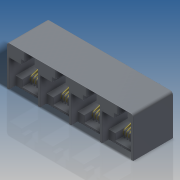
# Autodesk Inventor part: 11035-LtBluishGray
Saved by Autodesk Inventor 2016 SP2 (Build 200236200, 236)
## iProperties
Created: 2015-08-19
Part Number: 11035-LtBluishGray
Material: ABS Plastic
Document SubType Name: Modeling
Designer: D. Kohfeld
Density: 1.06 g/cm^3
Appearance: LtBluishGray
Mass: 4.59021 g
Surface Area: 62.0257 cm^2
Volume: 4.33039 cm^3
Author: D. Kohfeld
Autodesk Inventor part; units mm, degrees
ref_plane "XZ Plane" through (0, 0, 0) normal (0, 1, 0) x (-1, 0, 0)
ref_plane "XY Plane" through (0, 0, 0) normal (0, 0, 1) x (1, 0, 0)
sketch "Sketch2" plane through (0, 0, 0) normal (0, 0, 1) x (1, 0, 0)
  line L0 (-22.8, -6.8) -> (-22.8, 6.8)
  arc A0 (-21.84, 7.76) -> (-22.8, 6.8) centre (-21.84, 6.8) ccw
  line L1 (-21.84, 7.76) -> (21.84, 7.76)
  arc A1 (22.8, 6.8) -> (21.84, 7.76) centre (21.84, 6.8) ccw
  line L2 (22.8, 6.8) -> (22.8, -6.8)
  line L3 (22.8, -6.8) -> (-22.8, -6.8)
  line L4 (-22, -6.8) -> (-22, 3.2)
  line L5 (-22, 3.2) -> (-17.6, 3.2)
  line L6 (-17.6, 3.2) -> (-17.6, 4.8)
  line L7 (-17.6, 4.8) -> (-16.4, 4.8)
  line L8 (-16.4, 4.8) -> (-16.4, 6.8)
  line L9 (-16.4, 6.8) -> (-12.8, 6.8)
  line L10 (-12.8, 6.8) -> (-12.8, 4.8)
  line L11 (-12.8, 4.8) -> (-11.6, 4.8)
  line L12 (-11.6, 4.8) -> (-11.6, -6.8)
  line L13 (-22, -3.6) -> (-19.6, -3.6)
  line L14 (-19.6, -3.6) -> (-19.6, -6)
  line L15 (-19.6, -6) -> (-19, -6)
  line L16 (-19, -6) -> (-18.6, -6)
  line L17 (-18.6, -6) -> (-18, -6)
  line L18 (-18, -6) -> (-17.6, -6)
  line L19 (-17.6, -6) -> (-17, -6)
  line L20 (-17, -6) -> (-16.6, -6)
  line L21 (-16.6, -6) -> (-16, -6)
  line L22 (-16, -6) -> (-15.6, -6)
  line L23 (-15.6, -6) -> (-15, -6)
  line L24 (-15, -6) -> (-14.6, -6)
  line L25 (-14.6, -6) -> (-14, -6)
  line L26 (-14, -6) -> (-14, -3.6)
  line L27 (-14, -3.6) -> (-11.6, -3.6)
  line L28 (-19, -6) -> (-19, -3.6)
  line L29 (-18.6, -6) -> (-18.6, -3.6)
  line L30 (-18, -6) -> (-18, -3.6)
  line L31 (-17.6, -6) -> (-17.6, -3.6)
  line L32 (-17, -6) -> (-17, -3.6)
  line L33 (-16.6, -6) -> (-16.6, -3.6)
  line L34 (-16, -6) -> (-16, -3.6)
  line L35 (-15.6, -6) -> (-15.6, -3.6)
  line L36 (-15, -6) -> (-15, -3.6)
  line L37 (-14.6, -6) -> (-14.6, -3.6)
  line L38 (-19.6, -3.6) -> (-19, -3.6)
  line L39 (-19, -3.6) -> (-18.6, -3.6)
  line L40 (-18.6, -3.6) -> (-18, -3.6)
  line L41 (-18, -3.6) -> (-17.6, -3.6)
  line L42 (-17.6, -3.6) -> (-17, -3.6)
  line L43 (-17, -3.6) -> (-16.6, -3.6)
  line L44 (-16.6, -3.6) -> (-16, -3.6)
  line L45 (-16, -3.6) -> (-15.6, -3.6)
  line L46 (-15.6, -3.6) -> (-15, -3.6)
  line L47 (-15, -3.6) -> (-14.6, -3.6)
  line L48 (-14.6, -3.6) -> (-14, -3.6)
  line L49 (-17.6, 4.8) -> (-17.6, 6.8)
  line L50 (-17.6, 6.8) -> (-16.4, 6.8)
  line L51 (-12.8, 6.8) -> (-11.6, 6.8)
  line L52 (-11.6, 6.8) -> (-11.6, 4.8)
  point P0 (0, 0)
  point P1 (0, 7.76)
  point P2 (-22.8, 0)
  dimension "d0" = 45.6
  dimension "d1" = 14.56
  dimension "d2" = 0.96
  dimension "d3" = 10.4
  dimension "d4" = 0.96
  dimension "d5" = 3.6
  dimension "d6" = 6
  dimension "d8" = 2
  dimension "d9" = 1.6
  dimension "d10" = 0.8
  dimension "d11" = 3.2
  dimension "d12" = 2.4
  dimension "d13" = 0.4
  dimension "d14" = 5.6
  constraints: 106 end point, 32 horizontal, 21 vertical, 11 collinear, 4 point on circle, 4 point on line, 4 tangent, 2 centre point, 2 horizontal alignment, 2 midpoint, 1 equal radius, 1 vertical alignment
  measures "d0" distance between parallel lines of L0 L2
  measures "d1" distance between parallel lines of L3 L1
  measures "d2" radius of A0
  measures "d3" distance between parallel lines of L12 L4
  measures "d4" distance between parallel lines of L1 L9
  measures "d5" distance of L8.end L9.end
  measures "d6" distance between parallel lines of L12 L6
  measures "d8" distance of L7.end L8.end
  measures "d9" distance of L5.end L6.end
  measures "d10" distance between parallel lines of L0 L4
  measures "d11" distance between parallel lines of L3 L13
  measures "d12" distance of L13.end L14.end
  measures "d13" distance between parallel lines of L29 L28
  measures "d14" distance between parallel lines of L26 L14
extrude "Extrusion1" add sketch "Sketch2" against normal blind 14.4
extrude "Extrusion2" cut sketch "Sketch2" against normal blind 12.8 contours L4 L5 L6 L7 L8 L9 L10 L11 L12 L27 L48 L47 L46 L45 L44 L43 L42 L41 L40 L39 L38 L13 | L11 L10 L51 L52 | L49 L50 L8 L7
extrude "Extrusion3" add sketch "Sketch2" against normal blind 2.8 contours L11 L10 L51 L52 | L49 L50 L8 L7
extrude "Extrusion4" cut sketch "Sketch2" against normal blind 9.6 contours L38 L28 L15 L14 | L26 L25 L37 L48 | L40 L30 L17 L29 | L36 L23 L35 L46 | L42 L32 L19 L31 | L34 L21 L33 L44
extrude "Extrusion5" cut sketch "Sketch2" against normal blind 2.4 contours L4 L13 L14 L15 L16 L17 L18 L19 L20 L21 L22 L23 L24 L25 L26 L27 L12 L3 | L39 L29 L16 L28 | L37 L24 L36 L47 | L41 L31 L18 L30 | L35 L22 L34 L45 | L43 L33 L20 L32
extrude "Extrusion6" cut sketch "Sketch2" against normal blind 4.8 contours L39 L29 L16 L28 | L37 L24 L36 L47 | L41 L31 L18 L30 | L35 L22 L34 L45 | L43 L33 L20 L32
sketch "Sketch3" plane through (0, 0, -9.6) normal (0, 0, 1) x (1, 0, 0)
  line L0 (-19, -6) -> (-19.6, -6) projected
  circle A0 centre (-19.3, -5.71) radius 0.29
  line L1 (-19.6, -6) -> (-14, -6) projected
  point P0 (0, 0)
  point P1 (-19.3, -6)
  dimension "d27" = 0.58
  constraints: 1 centre point, 1 midpoint, 1 tangent, 1 vertical alignment
  measures "d27" diameter of A0
ref_plane "Work Plane1" through (-19.3, -5.71, -9.6) normal (1, 0, 0) x (0, 1, 0)
sketch "Sketch4" plane through (-19.3, -5.71, -9.6) normal (1, 0, 0) x (0, 1, 0)
  line L0 (-0.29, 4.8) -> (2.11, 4.8) projected
  line L1 (2.11, 0) -> (2.11, 4.8) projected
  line L2 (0, 0) -> (0, 3.51)
  arc A0 (1.9509, 3.8195) -> (0, 3.51) centre (1, 3.51) ccw
  line L3 (1.9509, 3.8195) -> (3.91, -2.2)
  line L4 (-0.29, 0) -> (2.11, 0) projected
  point P0 (5.71, 9.6)
  dimension "d28" = 0.29
  dimension "d29" = 1
  dimension "d31" = 1.8
  dimension "d32" = 2.2
  constraints: 4 end point, 2 point on circle, 2 tangent, 1 centre point, 1 vertical
  measures "d28" distance edge to line of A0 L0
  measures "d29" radius of A0
  measures "d31" distance from line of L3.end L1
  measures "d32" distance from line of L3.end L4
sweep "Sweep1" add profiles "Sketch3" path "Sketch4" path curves L2 A0 L3
pattern_linear "Rectangular Pattern1" count 6 spacing 1 along (1, 0, 0) of "Sweep1"
sketch "Sketch5" plane through (-16.4, 4.8, 0) normal (1, 0, 0) x (0, 0, -1)
  line L0 (0, 2) -> (2.8, 2) projected
  line L1 (0, 2) -> (0, 2.8)
  line L2 (0, 2.8) -> (2.8, 2)
  point P0 (0, -4.8)
  dimension "d37" = 0.8
  constraints: 4 end point, 1 vertical
  measures "d37" distance of L0.start L1.end
extrude "Extrusion7" cut sketch "Sketch5" along normal blind 3.6
fillet "Fillet1" radius 0.1 25 edges at (-20.8, -3.6, -2.4) (-19.6, -3.6, -6) (-19.6, -4.8, -2.4) (-16.8, -6, -2.4) (-18.8, -3.6, -4.8) (-17.8, -3.6, -4.8) (-16.8, -3.6, -4.8) (-15.8, -3.6, -4.8) (-14.8, -3.6, -4.8) (-12.8, -3.6, -2.4) (-14, -3.6, -6) (-14, -4.8, -2.4) (-11.6, -1, 0) (-12.2, 4.8, 0) (-12.8, 4.8, -1.4) (-12.8, 6.2, 0) (-14.6, 7.6, 0) (-16.4, 6.2, 0) (-17, 4.8, 0) (-16.4, 4.8, -1.4) (-17.6, 4, 0) (-17.6, 3.2, -6.4) (-19.8, 3.2, 0) (-22, -1.8, 0) (-14.6, 6.8, -2.8)
pattern_linear "Rectangular Pattern2" count 4 spacing 11.2 along (1, 0, 0) of "Extrusion2", "Extrusion3", "Extrusion4", "Extrusion5", "Extrusion6", "Extrusion7", "Fillet1"
pattern_linear "Rectangular Pattern3" count 4 spacing 11.2 along (1, 0, 0) of "Sweep1", "Rectangular Pattern1"
fillet "Fillet2" radius 0.1 38 edges at (-22.5188, 7.4788, 0) (-22.8, 0, 0) (22.5188, 7.4788, 0) (22.8, 0, 0) (0, 7.76, 0) (-22, -6.8, -1.25) (-22.45, -6.8, 0) (-22.0293, -6.8, -0.0293) (-10.8293, -6.8, -0.0293) (-10.8, -6.8, -1.25) (-11.5707, -6.8, -0.0293) (-11.6, -6.8, -1.25) (-11.2, -6.8, 0) (0.4, -6.8, -1.25) (0, -6.8, 0) (-0.3707, -6.8, -0.0293) (-0.4, -6.8, -1.25) (0.3707, -6.8, -0.0293) (11.5707, -6.8, -0.0293) (11.6, -6.8, -1.25) (10.8293, -6.8, -0.0293) (10.8, -6.8, -1.25) (11.2, -6.8, 0) (22.0293, -6.8, -0.0293) (22, -6.8, -1.25) (22.45, -6.8, 0) (22.8, -6.8, -7.2) (22.5188, 7.4788, -14.4) (0, 7.76, -14.4) (-22.5188, 7.4788, -14.4) (-22.8, 0, -14.4) (22.8, 0, -14.4) (0, -6.8, -14.4) (-16.8, -6.8, -2.4) (-5.6, -6.8, -2.4) (5.6, -6.8, -2.4) (16.8, -6.8, -2.4) (-22.8, -6.8, -7.2)
equation "\"d21\" = lh"
equation "\"d28\" = 0.5 * d27"
equation "\"lh\" = 9.6"
body "Solid1"
